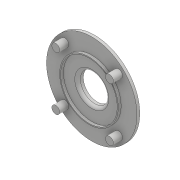
# Autodesk Inventor part: pot_base_adapter2
Saved by Autodesk Inventor 2017 (Build 210142000, 142)
## iProperties
Created: 2018-10-29
Part Number: pot_base_adapter2
Material: Generic
Document SubType Name: Modeling
Designer: mfans
Density: 1 g/cm^3
Appearance: Default
Author: mfans
Autodesk Inventor part; units mm, degrees
ref_plane "YZ Plane" through (0, 0, 0) normal (1, 0, 0) x (0, 1, 0)
ref_plane "XZ Plane" through (0, 0, 0) normal (0, 1, 0) x (-1, 0, 0)
ref_plane "XY Plane" through (0, 0, 0) normal (0, 0, 1) x (1, 0, 0)
sketch "Sketch1" plane through (0, 0, 0) normal (0, 1, 0) x (-1, 0, 0)
  circle A0 centre (0, 0) radius 32
  dimension "d0" = 64
  constraints: 1 centre point, 1 coincident
  measures "d0" diameter of A0
extrude "Extrusion1" add sketch "Sketch1" along normal blind 2
sketch "Sketch2" plane through (0, 0, 0) normal (0, -1, 0) x (1, 0, 0)
  circle A0 centre (0, 0) radius 20.75
  circle A1 centre (0, 0) radius 20
  dimension "d3" = 41.5
  dimension "d4" = 40
  constraints: 2 centre point, 2 coincident
  measures "d3" diameter of A0
  measures "d4" diameter of A1
extrude "Extrusion2" add sketch "Sketch2" along normal blind 2
sketch "Sketch4" plane through (0, 0, 0) normal (0, -1, 0) x (1, 0, 0)
  circle A0 centre (19, 19) radius 2.75
  point P0 (0, 0)
  dimension "d9" = 5.5
  dimension "d10" = 19
  dimension "d11" = 19
  constraints: 1 centre point
  measures "d9" diameter of A0
  measures "d10" horizontal distance of point (0, 0) A0.centre
  measures "d11" horizontal distance of point (0, 0) A0.centre
extrude "Extrusion4" add sketch "Sketch4" along normal blind 6.5
pattern_circular "Circular Pattern1" count 4 over 360 about axis through (0, -10, 0) along (0, 1, 0) of "Extrusion4"
sketch "Sketch5" plane through (0, 2, 0) normal (0, 1, 0) x (1, 0, 0)
  line L0 (-12.25, 12.25) -> (12.25, 12.25)
  line L1 (12.25, 12.25) -> (12.25, -12.25)
  line L2 (12.25, -12.25) -> (-12.25, -12.25)
  line L3 (-12.25, -12.25) -> (-12.25, 12.25)
  line L4 (-12.25, 12.25) -> (12.25, -12.25) construction
  line L5 (12.25, 12.25) -> (-12.25, -12.25) construction
  point P0 (0, 0)
  dimension "d17" = 24.5
  dimension "d18" = 24.5
  constraints: 12 end point, 2 midpoint, 2 parallel, 1 horizontal, 1 perpendicular
  measures "d17" distance of L1.end L2.end
  measures "d18" distance of L2.end L0.start
extrude "Extrusion5" add sketch "Sketch5" along normal blind 2
sketch "Sketch6" plane through (0, 4, 0) normal (0, 1, 0) x (1, 0, 0)
  line L0 (12.25, 12.25) -> (-12.25, 12.25) projected
  line L1 (-12.25, 12.25) -> (-12.25, -12.25) projected
  line L2 (-12.25, -12.25) -> (12.25, -12.25) projected
  line L3 (12.25, -12.25) -> (12.25, 12.25) projected
  circle A0 centre (0, 0) radius 10
  dimension "d21" = 20
  constraints: 1 centre point, 1 coincident
  measures "d21" diameter of A0
extrude "Extrusion6" cut sketch "Sketch6" against normal through all contours A0
fillet "Fillet1" radius 2 1 edges at (-10, 0, 0)
body "Solid1"
